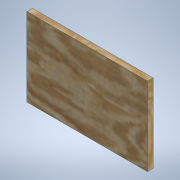
# Autodesk Inventor part: Side Piece
Saved by Autodesk Inventor 2020 (Build 240168000, 168)
## iProperties
Created: 2020-01-25
Part Number: Side Piece
Material: Wood (Oak)
Document SubType Name: Modeling
Designer: 1cikaychapman
Density: 0.76 g/cm^3
Appearance: Plywood - Weathered
Author: 1cikaychapman
Autodesk Inventor part; units mm, degrees
ref_plane "YZ Plane" through (0, 0, 0) normal (1, 0, 0) x (0, 1, 0)
ref_plane "XZ Plane" through (0, 0, 0) normal (0, 1, 0) x (-1, 0, 0)
ref_plane "XY Plane" through (0, 0, 0) normal (0, 0, 1) x (1, 0, 0)
sketch "Sketch1" plane through (0, 0, 0) normal (0, 0, 1) x (1, 0, 0)
  line L0 (0, 0) -> (273.05, 0)
  line L1 (273.05, 0) -> (273.05, 177.8)
  line L2 (273.05, 177.8) -> (0, 177.8)
  line L3 (0, 177.8) -> (0, 0)
  dimension "d0" = 273.05
  dimension "d1" = 177.8
  constraints: 8 end point, 2 parallel, 1 horizontal, 1 perpendicular
  measures "d0" distance of L2.end L1.end
  measures "d1" distance of L0.end L1.end
extrude "Extrusion1" add sketch "Sketch1" along normal blind 12.7
body "Solid1"
